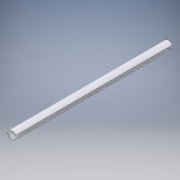
# Autodesk Inventor part: inner_sheath
Saved by Autodesk Inventor 2017 (Build 210142000, 142)
## iProperties
Created: 2018-11-30
Part Number: inner_sheath
Material: Acetal Resin, White
Document SubType Name: Modeling
Designer: ddeboer
Density: 1.425 g/cm^3
Appearance: Smooth - White
Author: ddeboer
Autodesk Inventor part; units mm, degrees
ref_plane "YZ Plane" through (0, 0, 0) normal (1, 0, 0) x (0, 1, 0)
ref_plane "XZ Plane" through (0, 0, 0) normal (0, 1, 0) x (-1, 0, 0)
ref_plane "XY Plane" through (0, 0, 0) normal (0, 0, 1) x (1, 0, 0)
sketch "Sketch1" plane through (0, 0, 0) normal (0, 0, 1) x (1, 0, 0)
  circle A0 centre (0, 0) radius 13.27
  circle A1 centre (0, 0) radius 10.325
  dimension "d0" = 26.54
  dimension "d1" = 20.65
  constraints: 2 centre point, 2 coincident
  measures "d0" diameter of A0
  measures "d1" diameter of A1
extrude "Extrusion1" add sketch "Sketch1" along normal blind 500
sketch "Sketch2" plane through (0, 0, 500) normal (0, 0, 1) x (1, 0, 0)
  line L0 (12.0196, -5.4434) -> (14.8291, -5.4434)
  line L1 (14.8291, -5.4434) -> (14.8291, 5.5566)
  line L2 (14.8291, 5.5566) -> (12.0196, 5.5566)
  line L3 (12.0196, 5.5566) -> (12.0196, -5.4434)
  point P0 (0, 0)
  dimension "d4" = 11
  constraints: 8 end point, 2 parallel, 1 horizontal, 1 perpendicular
  measures "d4" distance of L0.end L1.end
extrude "Extrusion2" cut sketch "Sketch2" against normal blind 500
sketch "Sketch3" plane through (12.0196, -5.4434, 500) normal (1, 0, 0) x (0, 0, -1)
  line L0 (0, -4.8816) -> (0, 15.7684) projected
  line L1 (0, 11) -> (500, 11) projected
  line L2 (0, -0.0645) -> (500, -0.0645)
  line L3 (500, -0.0645) -> (500, 11)
  line L4 (500, 11) -> (0, 11)
  line L5 (0, 11) -> (0, -0.0645)
  point P0 (500, 5.4434)
  constraints: 8 end point, 2 parallel, 1 horizontal, 1 perpendicular, 1 point on line
extrude "Extrusion3" cut sketch "Sketch3" against normal blind 10
ref_plane "Work Plane1" through (12.0506, 5.5566, 500) normal (0.999989, 0.0046908, 0) x (0.0046908, -0.999989, 0)
sketch "Sketch4" plane through (12.0506, 5.5566, 500) normal (0.999989, 0.0046908, 0) x (0.0046908, -0.999989, 0)
  circle A0 centre (5.5001, 475) radius 2
  point P0 (5.5001, 500)
  dimension "d9" = 25
  dimension "d10" = 4
  constraints: 1 centre point
  measures "d9" distance of point (5.5, 500) A0.centre
  measures "d10" diameter of A0
extrude "Extrusion4" cut sketch "Sketch4" against normal blind 40
body "Solid1"
